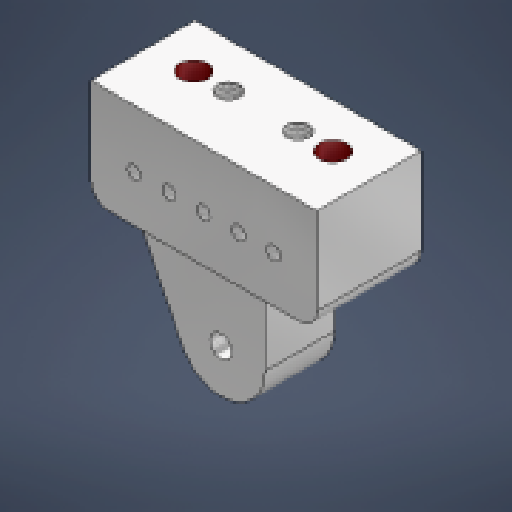
# Autodesk Inventor part: MOUNT,CHAIN,ELEVATOR
Saved by Autodesk Inventor 2024.3 (Build 283343000, 343)
## iProperties
ILogicPurgeVersion: 0.0.0.0
OnSaveVersion: 3.5.0.0
OnSaveAssembly: COREAutomationManager
Category: _
Manager: _
Created: 2025-03-04
Part Number: MOUNT,CHAIN,ELEVATOR
Checked By: 00
Engr Approved By: _
User Status: Work In Process
Material: Aluminum 7075
Description: STANDARD (mm)
Document SubType Name: Modeling
Mfg Approved By: John.Thibert
Designer: John.Thibert
Manufacturer: Standard
Standards Organization: Custom
Mass: 55.9634 g
Surface Area: 62.9161 cm^2
Volume: 19.9158 cm^3
Density: 2.81 g/cm^3
Appearance: Aluminum - Polished
CN_MASS: 0.06
CN_SERVICEABLE: _
FIRST_DESCRIPTION: _
SECOND_DESCRIPTION: _
THIRD_DESCRIPTION: _
ModelCat: Uncategorized
MaterialName: Aluminum 7075
Subject: _
Author: John.Thibert
Keywords: -
Revision Number: A
Autodesk Inventor part; units mm, degrees
ref_plane "YZ Plane" through (0, 0, 0) normal (1, 0, 0) x (0, 1, 0)
ref_plane "XZ Plane" through (0, 0, 0) normal (0, 1, 0) x (-1, 0, 0)
ref_plane "XY Plane" through (0, 0, 0) normal (0, 0, 1) x (1, 0, 0)
sketch "Sketch2" plane through (0, 0, 0) normal (0, 0, 1) x (1, 0, 0)
  line L0 (20.6375, 22.225) -> (-20.6375, 22.225)
  line L1 (-20.6375, 22.225) -> (-20.6375, -22.225) construction
  line L2 (-20.6375, -22.225) -> (20.6375, -22.225) construction
  line L3 (20.6375, -22.225) -> (20.6375, 22.225) construction
  line L4 (20.6375, 22.225) -> (-20.6375, -22.225) construction
  line L5 (-20.6375, 22.225) -> (20.6375, -22.225) construction
  line L6 (4.7625, -14.2875) -> (4.7625, 3.175)
  line L7 (4.7625, 3.175) -> (20.6375, 3.175)
  arc A0 (-10.293826, -17.798372) -> (4.7625, -14.2875) centre (-3.175, -14.2875) ccw
  line L8 (-20.6375, 3.175) -> (-10.293826, -17.798372)
  line L9 (20.6375, 3.175) -> (20.6375, 22.225)
  line L10 (-20.6375, 3.175) -> (-20.6375, 22.225)
  point P0 (0, 0)
  dimension "d0" = 41.275
  dimension "d1" = 44.45
  dimension "d4" = 19.05
  dimension "d8" = 15.875
  dimension "d10" = 25.4
  constraints: 22 end point, 3 point on line, 3 tangent, 2 collinear, 2 midpoint, 2 parallel, 2 perpendicular, 2 point on circle, 1 centre point, 1 horizontal, 1 vertical
  measures "d0" distance of L0.start L0.end
  measures "d1" distance of L0.end L1.end
  measures "d4" distance between parallel lines of L0 L7
  measures "d8" diameter of A0
  measures "d10" distance between parallel lines of L1 L6
extrude "Extrusion1" add sketch "Sketch2" along normal blind 19.05
fillet "Fillet1" radius 3.175 2 edges at (-20.6375, 3.175, 9.525) (4.7625, 3.175, 9.525)
sketch "Sketch3" plane through (-20.6375, 22.225, 0) normal (0, 1, 0) x (1, 0, 0)
  line L0 (7.9375, -8.189483) -> (33.3375, -8.189483) construction
  line L1 (41.275, 0) -> (0, 0) construction
  line L2 (0, 0) -> (0, -19.05) construction
  line L3 (41.275, 0) -> (41.275, -19.05) construction
  point P0 (20.6375, 0)
  point P1 (20.6375, 0)
  dimension "d11" = 8.18948
  dimension "d12" = 7.9375
  dimension "d13" = 7.9375
  dimension "d14" = 25.4
  constraints: 2 end point, 1 horizontal, 1 midpoint
  measures "d11" distance from line of point (20.638, 0) L0
  measures "d12" distance from line of L0.start L2
  measures "d13" distance from line of L3 L0.end
  measures "d14" distance of L0.start L0.end
hole "Hole1" at (-12.7, 22.225, 8.189483) at (12.7, 22.225, 8.189483) direction (0, -1, 0) diameter 5.0038 depth 6.35 tip angle 118 clearance for "H7 - STANDARD FIT" size "5" standard "CL-DOWEL-MET"
sketch "Sketch4" plane through (-20.6375, 22.225, 0) normal (0, 1, 0) x (1, 0, 0)
  circle A0 centre (7.9375, -8.189483) radius 2.5019 construction
  circle A1 centre (7.9375, -8.189483) radius 2.5019 construction
  circle A2 centre (33.3375, -8.189483) radius 2.5019 construction
  circle A3 centre (33.3375, -8.189483) radius 2.5019 construction
  line L0 (7.9375, -8.189483) -> (14.2875, -8.189483) construction
  line L1 (33.3375, -8.189483) -> (26.9875, -8.189483) construction
  point P0 (20.6375, 0)
  dimension "d22" = 6.35
  constraints: 4 end point, 2 horizontal, 1 collinear
  measures "d22" distance of L1.start L1.end
hole "Hole2" at (-6.35, 22.225, 8.189483) at (6.35, 22.225, 8.189483) direction (0, -1, 0) diameter 3.9624 depth 13.6144 tip angle 118 thread size "10-32 UNF" class "2B" standard "ANSI Unified Screw Threads"
sketch "Sketch5" plane through (0, 0, 0) normal (0, 0, -1) x (-1, 0, 0)
  arc A0 (-4.7625, -14.2875) -> (10.293826, -17.798372) centre (3.175, -14.2875) ccw construction
  point P0 (0, 0)
  constraints: 1 coincident
hole "Hole3" at (-3.175, -14.2875, 0) direction (0, 0, 1) diameter 3.9624 depth 13.6144 tip angle 118 thread size "10-32 UNF" class "2B" standard "ANSI Unified Screw Threads"
sketch "Sketch6" plane through (0, 0, 19.05) normal (0, 0, 1) x (1, 0, 0)
  arc A0 (-20.6375, 3.915354) -> (-20.31003, 2.511006) centre (-17.4625, 3.915354) ccw
  line L0 (-20.31003, 2.511006) -> (-10.293826, -17.798372)
  arc A1 (-10.293826, -17.798372) -> (4.7625, -14.2875) centre (-3.175, -14.2875) ccw
  line L1 (4.7625, -14.2875) -> (4.7625, 0)
  arc A2 (7.9375, 3.175) -> (4.7625, 0) centre (7.9375, 0) ccw
  line L2 (7.9375, 3.175) -> (20.6375, 3.175)
  line L3 (20.6375, 3.175) -> (20.6375, 22.225) construction
  line L4 (20.6375, 22.225) -> (-20.6375, 22.225) construction
  line L5 (-20.6375, 22.225) -> (-20.6375, 3.915354) construction
  line L6 (7.9375, 3.175) -> (-20.549975, 3.175)
  point P0 (0, 0)
  constraints: 2 end point, 1 horizontal, 1 point on circle, 1 tangent
extrude "Extrusion2" cut sketch "Sketch6" against normal blind 6.35
sketch "Sketch7" plane through (0, 0, 19.05) normal (0, 0, 1) x (1, 0, 0)
  line L0 (-20.6375, 22.225) -> (-20.6375, 3.915354) construction
  line L1 (20.6375, 3.175) -> (20.6375, 22.225) construction
  line L2 (-20.6375, 11.5951) -> (20.6375, 11.5951) construction
  line L3 (20.6375, 22.225) -> (-20.6375, 22.225) construction
  point P0 (0, 0)
  point P1 (0, 11.5951)
  dimension "d43" = 10.6299
  constraints: 2 end point, 2 point on line, 1 midpoint, 1 perpendicular
  measures "d43" distance between parallel lines of L3 L2
hole "Hole4" at (0, 11.5951, 19.05) direction (0, 0, -1) diameter 2.459 depth 12.7 tip angle 118 thread size "M3x0.5" class "6H" standard "ANSI Metric M Profile-Short lst"
pattern_linear "Rectangular Pattern1" count 5 spacing 6.35 along (1, 0, 0) of "Hole4" first direction both ways yes
fillet "Fillet3" radius 3.175 2 edges at (-20.55, 3.175, 15.875) (20.6375, 3.175, 9.525)
fillet "Fillet2" radius 3.175 1 edges at (-4.7625, 3.175, 12.7)
equation "\"d13\" = d12"
body "Solid1"
